Autodesk Fusion 360 part; units mm, degrees
(part 3 of 4)
  spline S1 degree 5 poles (46.7219, 69.0368) (46.744, 69.0368) (46.7882, 69.0364) (46.8546, 69.0344) (46.9431, 69.0291) (47.0539, 69.0189) (47.1646, 69.0061) (47.2752, 68.9921) (47.3856, 68.9776) (47.4957, 68.9631) (47.6056, 68.9482) (47.7152, 68.9327) (47.8246, 68.9161) (47.9339, 68.898) (48.043, 68.8784) (48.152, 68.8576) (48.2609, 68.8359) (48.3697, 68.8134) (48.4783, 68.7905) (48.5868, 68.7667) (48.6949, 68.742) (48.8027, 68.7157) (48.9099, 68.6877) (49.0166, 68.6578) (49.1229, 68.6261) (49.2287, 68.5929) (49.3342, 68.5585) (49.4395, 68.5233) (49.5445, 68.4876) (49.6493, 68.4511) (49.7537, 68.4138) (49.8576, 68.3753) (49.961, 68.3353) (50.0637, 68.2936) (50.1658, 68.2503) (50.2671, 68.2053) (50.3679, 68.159) (50.4681, 68.1114) (50.5678, 68.0629) (50.667, 68.0133) (50.7656, 67.9628) (50.8638, 67.9113) (50.9613, 67.8586) (51.0583, 67.8047) (51.1545, 67.7494) (51.2499, 67.6928) (51.3444, 67.6346) (51.438, 67.575) (51.5307, 67.5139) (51.6224, 67.4515) (51.7133, 67.3878) (51.8034, 67.3231) (51.8928, 67.2574) (51.9817, 67.1909) (52.07, 67.1238) (52.1579, 67.0561) (52.2454, 66.9877) (52.3323, 66.9187) (52.4188, 66.849) (52.5045, 66.7785) (52.5894, 66.707) (52.6733, 66.6343) (52.7562, 66.5605) (52.8379, 66.4854) (52.9186, 66.4092) (52.9985, 66.3321) (53.0777, 66.2544) (53.1565, 66.176) (53.2347, 66.0972) (53.3124, 66.0177) (53.3892, 65.9375) (53.4649, 65.8564) (53.5393, 65.7741) (53.6123, 65.6905) (53.684, 65.6058) (53.7546, 65.5202) (53.8243, 65.4337) (53.8933, 65.3467) (53.9617, 65.2592) (54.0293, 65.1712) (54.0961, 65.0826) (54.1618, 64.9932) (54.2262, 64.9028) (54.2891, 64.8115) (54.3506, 64.7192) (54.411, 64.626) (54.4703, 64.5322) (54.5289, 64.4379) (54.5866, 64.3432) (54.6436, 64.248) (54.6995, 64.1522) (54.7542, 64.0558) (54.8075, 63.9585) (54.8592, 63.8604) (54.9096, 63.7616) (54.9587, 63.6621) (55.0069, 63.5621) (55.0542, 63.4617) (55.1009, 63.3611) (55.1469, 63.2602) (55.192, 63.159) (55.236, 63.0573) (55.2787, 62.955) (55.3201, 62.8521) (55.3602, 62.7487) (55.399, 62.6447) (55.4367, 62.5404) (55.4734, 62.4357) (55.5094, 62.3308) (55.5446, 62.2257) (55.579, 62.1203) (55.6128, 62.0147) (55.6463, 61.9089) (55.6802, 61.8032) (55.7155, 61.698) (55.7535, 61.5938) (55.7954, 61.4912) (55.8424, 61.3909) (55.8953, 61.2935) (55.9545, 61.1995) (56.0198, 61.1093) (56.0911, 61.0234) (56.1677, 60.9421) (56.2492, 60.8658) (56.335, 60.7948) (56.4249, 60.7292) (56.5184, 60.6692) (56.6151, 60.6148) (56.7146, 60.5659) (56.8165, 60.522) (56.9203, 60.4826) (57.0255, 60.447) (57.1317, 60.4143) (57.2385, 60.3836) (57.3454, 60.3539) (57.4522, 60.3241) (57.5587, 60.2934) (57.6647, 60.261) (57.77, 60.2265) (57.8747, 60.1898) (57.9786, 60.151) (58.082, 60.1103) (58.1847, 60.0683) (58.2869, 60.025) (58.3886, 59.9809) (58.4898, 59.9358) (58.5907, 59.89) (58.6912, 59.8432) (58.7913, 59.7956) (58.8911, 59.7472) (58.9906, 59.6981) (59.0898, 59.6481) (59.1886, 59.5974) (59.2869, 59.5458) (59.3846, 59.4932) (59.4815, 59.4394) (59.5776, 59.384) (59.6727, 59.3271) (59.7668, 59.2686) (59.8601, 59.2086) (59.9527, 59.1475) (60.0447, 59.0854) (60.1363, 59.0227) (60.2275, 58.9593) (60.3182, 58.8952) (60.408, 58.8301) (60.4969, 58.7637) (60.5846, 58.6958) (60.671, 58.6263) (60.7563, 58.5554) (60.8407, 58.4833) (60.9244, 58.4104) (61.0078, 58.3369) (61.0907, 58.263) (61.1732, 58.1886) (61.2549, 58.1134) (61.3355, 58.0371) (61.4148, 57.9595) (61.4926, 57.8805) (61.5692, 57.8002) (61.6448, 57.7189) (61.7196, 57.6368) (61.7939, 57.5542) (61.868, 57.4714) (61.9414, 57.3881) (62.0141, 57.3042) (62.0857, 57.2193) (62.1557, 57.1334) (62.2242, 57.0461) (62.2911, 56.9576) (62.3567, 56.868) (62.4212, 56.7776) (62.485, 56.6867) (62.548, 56.5953) (62.6104, 56.5034) (62.6717, 56.411) (62.7319, 56.3178) (62.7906, 56.2237) (62.8478, 56.1287) (62.9035, 56.0327) (62.9579, 55.936) (63.0112, 55.8387) (63.0638, 55.741) (63.1157, 55.643) (63.1669, 55.5448) (63.2174, 55.4461) (63.2669, 55.347) (63.3153, 55.2472) (63.3623, 55.1468) (63.4079, 55.0456) (63.452, 54.9438) (63.4946, 54.8413) (63.5358, 54.7383) (63.5757, 54.6349) (63.6146, 54.5311) (63.6527, 54.427) (63.6901, 54.3227) (63.7269, 54.2181) (63.7631, 54.1132) (63.7982, 54.0079) (63.832, 53.9022) (63.8641, 53.796) (63.894, 53.6892) (63.9217, 53.5819) (63.9475, 53.474) (63.9717, 53.3657) (63.9947, 53.2571) (64.0171, 53.1484) (64.039, 53.0396) (64.0604, 52.9307) (64.0811, 52.8217) (64.1009, 52.7126) (64.1193, 52.6032) (64.1362, 52.4936) (64.1516, 52.3838) (64.1657, 52.2737) (64.1787, 52.1635) (64.1908, 52.0532) (64.2021, 51.9428) (64.2127, 51.8323) (64.2225, 51.7217) (64.2314, 51.611) (64.239, 51.5002) (64.2451, 51.3893) (64.2493, 51.2783) (64.2514, 51.1672) (64.2511, 51.0562) (64.2484, 50.9452) (64.2435, 50.8344) (64.2367, 50.7236) (64.2288, 50.6129) (64.2204, 50.5022) (64.2119, 50.3915) (64.2035, 50.2807) (64.195, 50.17) (64.1859, 50.0593) (64.1756, 49.9488) (64.1635, 49.8385) (64.1493, 49.7285) (64.1329, 49.6187) (64.1147, 49.5092) (64.0951, 49.3999) (64.0745, 49.2908) (64.0531, 49.1818) (64.0311, 49.073) (64.0084, 48.9644) (63.9846, 48.856) (63.9597, 48.748) (63.9332, 48.6402) (63.9052, 48.5328) (63.8756, 48.4259) (63.8445, 48.3194) (63.8118, 48.2135) (63.7778, 48.1079) (63.7427, 48.0028) (63.7065, 47.898) (63.6695, 47.7935) (63.6318, 47.6892) (63.5932, 47.5852) (63.5537, 47.4816) (63.513, 47.3784) (63.4708, 47.2758) (63.4271, 47.1739) (63.3816, 47.0727) (63.3346, 46.9722) (63.2863, 46.8723) (63.2368, 46.7729) (63.1866, 46.6739) (63.1356, 46.5753) (63.0839, 46.4771) (63.0314, 46.3793) (62.978, 46.2822) (62.9234, 46.1856) (62.8676, 46.0898) (62.8107, 45.9946) (62.7527, 45.9001) (62.6937, 45.8062) (62.6338, 45.7127) (62.573, 45.6198) (62.5112, 45.5276) (62.4483, 45.4361) (62.3842, 45.3456) (62.3186, 45.2561) (62.2515, 45.1677) (62.1831, 45.0803) (62.1136, 44.9938) (62.0431, 44.908) (61.9718, 44.8228) (61.8997, 44.7383) (61.8267, 44.6547) (61.7525, 44.572) (61.6771, 44.4907) (61.6004, 44.4105) (61.5227, 44.3311) (61.445, 44.2518) (61.3683, 44.1715) (61.2938, 44.0892) (61.2229, 44.0038) (61.1565, 43.9146) (61.0957, 43.8215) (61.0409, 43.7246) (60.9925, 43.6242) (60.9507, 43.521) (60.9156, 43.4154) (60.8872, 43.3079) (60.8653, 43.1989) (60.8499, 43.0889) (60.8409, 42.9781) (60.8381, 42.8669) (60.8415, 42.7557) (60.851, 42.6449) (60.8662, 42.5348) (60.8867, 42.4256) (60.9115, 42.3173) (60.9392, 42.2098) (60.968, 42.1026) (60.9964, 41.9954) (61.023, 41.8879) (61.047, 41.7797) (61.0685, 41.671) (61.0879, 41.5617) (61.106, 41.452) (61.1236, 41.3423) (61.141, 41.2325) (61.1582, 41.1228) (61.1746, 41.013) (61.1896, 40.9031) (61.2024, 40.793) (61.2128, 40.6826) (61.2208, 40.5719) (61.2269, 40.461) (61.2316, 40.3499) (61.2355, 40.2389) (61.239, 40.1278) (61.2421, 40.0168) (61.2445, 39.9058) (61.246, 39.7949) (61.2462, 39.6839) (61.2449, 39.573) (61.2421, 39.462) (61.2379, 39.351) (61.2325, 39.2401) (61.226, 39.1292) (61.2187, 39.0184) (61.2105, 38.9078) (61.2013, 38.7971) (61.1911, 38.6866) (61.1797, 38.5762) (61.1669, 38.466) (61.1527, 38.3559) (61.1368, 38.246) (61.1194, 38.1363) (61.1004, 38.0269) (61.0798, 37.9179) (61.0578, 37.8092) (61.0344, 37.7008) (61.0096, 37.5927) (60.9836, 37.4848) (60.9564, 37.3773) (60.928, 37.27) (60.8983, 37.1631) (60.8673, 37.0566) (60.8349, 36.9505) (60.8013, 36.8449) (60.7664, 36.7397) (60.7305, 36.6348) (60.6937, 36.5302) (60.6561, 36.4258) (60.6176, 36.3218) (60.5782, 36.2181) (60.5377, 36.1148) (60.4958, 36.0121) (60.4524, 35.9101) (60.4074, 35.8088) (60.361, 35.7081) (60.3132, 35.6081) (60.2643, 35.5086) (60.2146, 35.4095) (60.1642, 35.3108) (60.113, 35.2125) (60.061, 35.1145) (60.0081, 35.0171) (59.954, 34.9203) (59.8987, 34.8242) (59.842, 34.7288) (59.784, 34.6342) (59.7248, 34.5403) (59.6643, 34.4473) (59.6026, 34.355) (59.5397, 34.2635) (59.4757, 34.1728) (59.4105, 34.083) (59.3442, 33.994) (59.2768, 33.9058) (59.2083, 33.8185) (59.1388, 33.732) (59.0682, 33.6463) (58.9966, 33.5614) (58.9242, 33.4773) (58.8509, 33.394) (58.7768, 33.3113) (58.7018, 33.2294) (58.6261, 33.1482) (58.5496, 33.0677) (58.4723, 32.988) (58.3941, 32.9092) (58.315, 32.8314) (58.2349, 32.7545) (58.1538, 32.6787) (58.0717, 32.6039) (57.9887, 32.5302) (57.9048, 32.4575) (57.82, 32.3858) (57.7344, 32.3151) (57.6479, 32.2455) (57.5605, 32.177) (57.4723, 32.1096) (57.3832, 32.0435) (57.2934, 31.9785) (57.2027, 31.9146) (57.1115, 31.8514) (57.0198, 31.7889) (56.9277, 31.727) (56.8352, 31.6656) (56.7422, 31.605) (56.6487, 31.5453) (56.5544, 31.4868) (56.4594, 31.4297) (56.3634, 31.3742) (56.2666, 31.3202) (56.1691, 31.2675) (56.071, 31.2158) (55.9724, 31.165) (55.8735, 31.1149) (55.7742, 31.0657) (55.6743, 31.0176) (55.5738, 30.9708) (55.4727, 30.9256) (55.3707, 30.8821) (55.268, 30.8403) (55.1647, 30.7999) (55.0609, 30.7608) (54.9568, 30.7227) (54.8524, 30.6853) (54.7478, 30.6484) (54.643, 30.612) (54.5382, 30.576) (54.4331, 30.5405) (54.3277, 30.5058) (54.2221, 30.472) (54.116, 30.4396) (54.0094, 30.4089) (53.9022, 30.3803) (53.7945, 30.3537) (53.6863, 30.3292) (53.5777, 30.3064) (53.4688, 30.2852) (53.3596, 30.2651) (53.2504, 30.2459) (53.141, 30.2274) (53.0315, 30.2097) (52.9218, 30.1927) (52.812, 30.1767) (52.702, 30.1617) (52.5918, 30.1482) (52.4813, 30.1362) (52.3708, 30.1261) (52.2601, 30.1179) (52.1493, 30.1117) (52.0384, 30.1071) (51.9274, 30.1038) (51.8164, 30.1015) (51.7053, 30.0998) (51.5943, 30.0988) (51.4832, 30.0986) (51.3721, 30.0996) (51.2612, 30.102) (51.1503, 30.1063) (51.0396, 30.1124) (50.9289, 30.1203) (50.8183, 30.1293) (50.7077, 30.1392) (50.5971, 30.1495) (50.4865, 30.1602) (50.3761, 30.1715) (50.2658, 30.1842) (50.1558, 30.1989) (50.0462, 30.2162) (49.9371, 30.2363) (49.8284, 30.2591) (49.7203, 30.2841) (49.6126, 30.3107) (49.5052, 30.3382) (49.3979, 30.3658) (49.2906, 30.393) (49.183, 30.4195) (49.075, 30.4448) (48.9663, 30.4684) (48.8569, 30.4893) (48.7469, 30.5065) (48.6363, 30.5186) (48.5256, 30.5242) (48.4148, 30.5224) (48.3045, 30.5124) (48.195, 30.4943) (48.0865, 30.4685) (47.9797, 30.4359) (47.8747, 30.3971) (47.7721, 30.353) (47.6723, 30.3037) (47.5755, 30.2494) (47.482, 30.1902) (47.3918, 30.1263) (47.3048, 30.058) (47.2205, 29.986) (47.1382, 29.9113) (47.0572, 29.835) (46.9768, 29.758) (46.8963, 29.6812) (46.8152, 29.6052) (46.7333, 29.5304) (46.6504, 29.4567) (46.5663, 29.3844) (46.4812, 29.3132) (46.3951, 29.2433) (46.308, 29.1744) (46.2201, 29.1066) (46.1313, 29.0398) (46.0419, 28.974) (45.9517, 28.9092) (45.8608, 28.8456) (45.7691, 28.7831) (45.6767, 28.7218) (45.5834, 28.6618) (45.4894, 28.6029) (45.3947, 28.5451) (45.2994, 28.4883) (45.2035, 28.4325) (45.107, 28.3777) (45.01, 28.3239) (44.9123, 28.2714) (44.814, 28.2203) (44.7151, 28.1705) (44.6154, 28.1221) (44.5152, 28.0749) (44.4145, 28.0287) (44.3134, 27.9832) (44.212, 27.9383) (44.1103, 27.8939) (44.0084, 27.8502) (43.906, 27.8074) (43.8032, 27.766) (43.6997, 27.7262) (43.5956, 27.6882) (43.4909, 27.6518) (43.3856, 27.6169) (43.28, 27.5832) (43.174, 27.5504) (43.0678, 27.5185) (42.9613, 27.4875) (42.8545, 27.4576) (42.7474, 27.429) (42.6398, 27.402) (42.5318, 27.3767) (42.4234, 27.3531) (42.3146, 27.3311) (42.2056, 27.3106) (42.0963, 27.2912) (41.9869, 27.2727) (41.8775, 27.255) (41.7679, 27.2376) (41.6583, 27.2207) (41.5486, 27.2041) (41.4387, 27.1881) (41.3286, 27.173) (41.2184, 27.1594) (41.1081, 27.1478) (40.9975, 27.1384) (40.8868, 27.1314) (40.7759, 27.1266) (40.6649, 27.1235) (40.5538, 27.1216) (40.4427, 27.1205) (40.3316, 27.1199) (40.2205, 27.12) (40.1095, 27.1209) (39.9986, 27.1232) (39.8877, 27.1272) (39.7769, 27.1331) (39.6662, 27.1408) (39.5556, 27.15) (39.4451, 27.1603) (39.3346, 27.1714) (39.2242, 27.1832) (39.1139, 27.1956) (39.0036, 27.2088) (38.8936, 27.2231) (38.7837, 27.2389) (38.6741, 27.2563) (38.5647, 27.2754) (38.4557, 27.2963) (38.347, 27.3188) (38.2386, 27.3427) (38.1306, 27.3679) (38.0228, 27.394) (37.9152, 27.4209) (37.8078, 27.4484) (37.7004, 27.4764) (37.5932, 27.505) (37.4863, 27.5344) (37.3796, 27.565) (37.2735, 27.5972) (37.168, 27.6313) (37.0632, 27.6673) (36.959, 27.7053) (36.8555, 27.745) (36.7524, 27.7861) (36.6498, 27.8282) (36.5475, 27.8712) (36.4455, 27.915) (36.344, 27.9596) (36.2429, 28.0052) (36.1423, 28.0518) (36.0423, 28.0997) (35.9429, 28.1489) (35.8441, 28.1993) (35.7459, 28.2509) (35.6483, 28.3035) (35.5512, 28.3571) (35.4546, 28.4116) (35.3585, 28.4669) (35.2627, 28.523) (35.1674, 28.5799) (35.0726, 28.6376) (34.9785, 28.6964) (34.8851, 28.7564) (34.7927, 28.8178) (34.7013, 28.8807) (34.611, 28.9451) (34.5217, 29.0109) (34.4332, 29.078) (34.3456, 29.1461) (34.2585, 29.215) (34.172, 29.2846) (34.086, 29.3549) (34.0008, 29.4261) (33.9165, 29.4983) (33.8332, 29.5716) (33.7509, 29.6461) (33.6697, 29.7218) (33.5895, 29.7986) (33.5103, 29.8764) (33.4318, 29.955) (33.3541, 30.0343) (33.2772, 30.1144) (33.201, 30.1951) (33.1257, 30.2767) (33.0514, 30.3591) (32.9781, 30.4425) (32.9059, 30.5268) (32.8348, 30.6121) (32.7648, 30.6983) (32.696, 30.7855) (32.6283, 30.8735) (32.5617, 30.9622) (32.4961, 31.0518) (32.4315, 31.142) (32.3679, 31.233) (32.3053, 31.3246) (32.2437, 31.4168) (32.1831, 31.5098) (32.1237, 31.6035) (32.0655, 31.698) (32.0086, 31.7933) (31.9529, 31.8893) (31.8987, 31.9861) (31.8457, 32.0836) (31.794, 32.1818) (31.7435, 32.2806) (31.6941, 32.3799) (31.6455, 32.4796) (31.5977, 32.5796) (31.5505, 32.68) (31.5038, 32.7805) (31.4578, 32.8814) (31.4125, 32.9826) (31.3681, 33.0843) (31.3249, 33.1866) (31.2832, 33.2895) (31.2432, 33.3931) (31.2053, 33.4974) (31.1696, 33.6025) (31.1361, 33.7081) (31.1044, 33.8143) (31.0739, 33.9209) (31.0439, 34.0277) (31.0133, 34.1343) (30.9811, 34.2406) (30.9464, 34.3461) (30.9083, 34.4505) (30.866, 34.5533) (30.8192, 34.6539) (30.7675, 34.752) (30.7105, 34.8472) (30.6482, 34.939) (30.5807, 35.0273) (30.5081, 35.1116) (30.4306, 35.1918) (30.3484, 35.2673) (30.2618, 35.3377) (30.1712, 35.4024) (30.0768, 35.461) (29.979, 35.5134) (29.8783, 35.5598) (29.7752, 35.6007) (29.6703, 35.6372) (29.5642, 35.6702) (29.4573, 35.7012) (29.3503, 35.7312) (29.2435, 35.7612) (29.137, 35.7921) (29.0311, 35.8245) (28.9258, 35.8588) (28.8212, 35.8952) (28.7172, 35.9336) (28.6138, 35.9738) (28.511, 36.0156) (28.4087, 36.0586) (28.3068, 36.1025) (28.2053, 36.1473) (28.1042, 36.1928) (28.0035, 36.2392) (27.9033, 36.2865) (27.8036, 36.3348) (27.7044, 36.3842) (27.6058, 36.4349) (27.5078, 36.4868) (27.4106, 36.5399) (27.3139, 36.5943) (27.2179, 36.6499) (27.1225, 36.7064) (27.0275, 36.7638) (26.933, 36.822) (26.8389, 36.8809) (26.7453, 36.9406) (26.6524, 37.0012) (26.5602, 37.063) (26.4688, 37.126) (26.3784, 37.1904) (26.289, 37.256) (26.2003, 37.3228) (26.1125, 37.3907) (26.0254, 37.4595) (25.9389, 37.5292) (25.8532, 37.5997) (25.7682, 37.6711) (25.6839, 37.7434) (25.6006, 37.8168) (25.5182, 37.8912) (25.4368, 37.9666) (25.3563, 38.0431) (25.2767, 38.1205) (25.1981, 38.1989) (25.1202, 38.2781) (25.0433, 38.3581) (24.9672, 38.4389) (24.8919, 38.5205) (24.8174, 38.6028) (24.7437, 38.6858) (24.6709, 38.7696) (24.5988, 38.854) (24.5276, 38.9392) (24.4572, 39.0251) (24.3877, 39.1117) (24.3193, 39.1992) (24.252, 39.2875) (24.1859, 39.3766) (24.1211, 39.4667) (24.0577, 39.5577) (23.9954, 39.6496) (23.9343, 39.7421) (23.8741, 39.8353) (23.8148, 39.9291) (23.7563, 40.0234) (23.6988, 40.1182) (23.6425, 40.2137) (23.5874, 40.31) (23.5337, 40.407) (23.4816, 40.505) (23.4309, 40.6037) (23.3815, 40.7031) (23.3332, 40.803) (23.2857, 40.9033) (23.2391, 41.004) (23.1933, 41.105) (23.1486, 41.2064) (23.105, 41.3083) (23.0626, 41.4107) (23.0216, 41.5136) (22.9817, 41.6171) (22.9427, 41.7209) (22.9045, 41.8251) (22.8669, 41.9295) (22.8299, 42.0342) (22.7938, 42.1391) (22.7591, 42.2444) (22.726, 42.3502) (22.6951, 42.4566) (22.6663, 42.5637) (22.6396, 42.6713) (22.6146, 42.7794) (22.5909, 42.8879) (22.568, 42.9966) (22.5459, 43.1053) (22.5245, 43.2142) (22.5039, 43.3232) (22.4846, 43.4324) (22.4667, 43.5418) (22.4504, 43.6515) (22.4359, 43.7615) (22.4229, 43.8717) (22.4113, 43.9821) (22.4009, 44.0926) (22.3914, 44.2032) (22.3826, 44.3138) (22.3747, 44.4246) (22.3674, 44.5353) (22.361, 44.6462) (22.3557, 44.7572) (22.3519, 44.8682) (22.3499, 44.9792) (22.3499, 45.0903) (22.3523, 45.2012) (22.3569, 45.3121) (22.3632, 45.4229) (22.3708, 45.5337) (22.3789, 45.6444) (22.3871, 45.7551) (22.3951, 45.8659) (22.4031, 45.9766) (22.4116, 46.0873) (22.4211, 46.1979) (22.4323, 46.3083) (22.4457, 46.4185) (22.4613, 46.5285) (22.4791, 46.6381) (22.499, 46.7473) (22.5206, 46.8562) (22.5436, 46.9648) (22.5677, 47.0731) (22.5928, 47.1812) (22.6186, 47.289) (22.6451, 47.3967) (22.6723, 47.5043) (22.7004, 47.6116) (22.7294, 47.7187) (22.7597, 47.8254) (22.7914, 47.9318) (22.8246, 48.0376) (22.8594, 48.1429) (22.8956, 48.2478) (22.9333, 48.3521) (22.9722, 48.4559) (23.0123, 48.5593) (23.0535, 48.6623) (23.0957, 48.7648) (23.139, 48.8669) (23.1834, 48.9686) (23.2289, 49.0698) (23.2756, 49.1704) (23.3236, 49.2705) (23.3729, 49.3699) (23.4236, 49.4685) (23.4757, 49.5665) (23.5289, 49.6638) (23.5833, 49.7604) (23.6386, 49.8565) (23.6947, 49.9522) (23.7516, 50.0474) (23.8092, 50.1422) (23.8677, 50.2364) (23.9272, 50.3301) (23.9877, 50.4231) (24.0495, 50.5152) (24.1126, 50.6065) (24.1771, 50.6969) (24.2429, 50.7863) (24.3099, 50.8747) (24.3781, 50.9623) (24.4471, 51.0492) (24.5168, 51.1355) (24.587, 51.2215) (24.6576, 51.3072) (24.7287, 51.3924) (24.8006, 51.4769) (24.8738, 51.5603) (24.9487, 51.6423) (25.0254, 51.7227) (25.1034, 51.802) (25.1817, 51.881) (25.2591, 51.9608) (25.3339, 52.0428) (25.4046, 52.128) (25.4701, 52.2173) (25.5299, 52.3108) (25.5835, 52.4083) (25.6312, 52.5092) (25.6729, 52.6128) (25.7087, 52.7186) (25.7384, 52.8259) (25.7617, 52.9345) (25.7784, 53.0441) (25.788, 53.1545) (25.7907, 53.2654) (25.7868, 53.3765) (25.7767, 53.4874) (25.7614, 53.5977) (25.7416, 53.7074) (25.7185, 53.8161) (25.693, 53.9242) (25.6661, 54.0317) (25.6387, 54.139) (25.6117, 54.2465) (25.5859, 54.3543) (25.5618, 54.4626) (25.5399, 54.5714) (25.5201, 54.6807) (25.5027, 54.7904) (25.4873, 54.9003) (25.4735, 55.0104) (25.4607, 55.1207) (25.4484, 55.231) (25.4361, 55.3413) (25.4238, 55.4516) (25.4118, 55.562) (25.4007, 55.6725) (25.3913, 55.783) (25.384, 55.8937) (25.3792, 56.0045) (25.3766, 56.1155) (25.3758, 56.2265) (25.3762, 56.3376) (25.3772, 56.4487) (25.3786, 56.5599) (25.3805, 56.6709) (25.3834, 56.7819) (25.3877, 56.8928) (25.3941, 57.0035) (25.4027, 57.1141) (25.4136, 57.2246) (25.4264, 57.3349) (25.4407, 57.4451) (25.456, 57.5551) (25.4719, 57.6649) (25.4881, 57.7747) (25.5045, 57.8843) (25.5213, 57.994) (25.5387, 58.1035) (25.5568, 58.213) (25.5763, 58.3223) (25.5973, 58.4313) (25.6204, 58.5398) (25.6456, 58.6478) (25.6731, 58.7552) (25.7025, 58.8621) (25.7334, 58.9686) (25.7655, 59.0748) (25.7982, 59.1808) (25.8314, 59.2867) (25.8652, 59.3923) (25.8998, 59.4977) (25.9357, 59.6025) (25.9732, 59.7068) (26.0123, 59.8105) (26.0531, 59.9136) (26.0951, 60.0162) (26.1381, 60.1185) (26.1816, 60.2205) (26.2257, 60.3224) (26.2703, 60.424) (26.3157, 60.5252) (26.3624, 60.6258) (26.4105, 60.7257) (26.4603, 60.8247) (26.5118, 60.9229) (26.5648, 61.0204) (26.6191, 61.1172) (26.6744, 61.2135) (26.7305, 61.3092) (26.7875, 61.4045) (26.8454, 61.4991) (26.9043, 61.5931) (26.9645, 61.6863) (27.0259, 61.7787) (27.0886, 61.8702) (27.1525, 61.9609) (27.2176, 62.0508) (27.2838, 62.1399) (27.351, 62.2283) (27.4192, 62.3159) (27.4886, 62.4026) (27.559, 62.4884) (27.6306, 62.5732) (27.7034, 62.657) (27.7772, 62.7399) (27.852, 62.8219) (27.9277, 62.9032) (28.0041, 62.9838) (28.0811, 63.0637) (28.1588, 63.1431) (28.237, 63.2218) (28.316, 63.2999) (28.3957, 63.3771) (28.4762, 63.4536) (28.5576, 63.529) (28.64, 63.6035) (28.7234, 63.6768) (28.8079, 63.7489) (28.8933, 63.8198) (28.9798, 63.8893) (29.0673, 63.9577) (29.1557, 64.0248) (29.245, 64.0907) (29.3351, 64.1555) (29.4258, 64.2194) (29.5171, 64.2824) (29.6089, 64.3447) (29.7011, 64.4063) (29.7938, 64.4674) (29.8869, 64.5277) (29.9804, 64.5873) (30.0746, 64.646) (30.1694, 64.7036) (30.2649, 64.7601) (30.3611, 64.8152) (30.4582, 64.8688) (30.5561, 64.9208) (30.6549, 64.9713) (30.7543, 65.0202) (30.8545, 65.0677) (30.9552, 65.114) (31.0564, 65.1592) (31.158, 65.2037) (31.2599, 65.2473) (31.3622, 65.2902) (31.4649, 65.3321) (31.568, 65.3728) (31.6716, 65.4124) (31.7757, 65.4507) (31.8802, 65.4877) (31.9851, 65.5236) (32.0903, 65.5585) (32.1958, 65.5926) (32.3015, 65.6259) (32.4075, 65.6583) (32.5139, 65.6897) (32.6206, 65.7198) (32.7277, 65.7485) (32.8353, 65.7757) (32.9433, 65.8011) (33.0517, 65.8248) (33.1605, 65.8467) (33.2696, 65.8671) (33.3788, 65.8861) (33.4883, 65.904) (33.5979, 65.9209) (33.7076, 65.9372) (33.8175, 65.9529) (33.9274, 65.968) (34.0376, 65.9821) (34.1478, 65.9948) (34.2583, 66.0057) (34.3689, 66.0144) (34.4797, 66.0206) (34.5907, 66.0247) (34.7017, 66.0268) (34.8128, 66.0276) (34.9238, 66.0275) (35.0349, 66.0269) (35.1459, 66.026) (35.2568, 66.025) (35.3678, 66.0237) (35.4789, 66.0219) (35.5899, 66.0193) (35.7009, 66.0155) (35.8118, 66.0102) (35.9226, 66.0029) (36.0331, 65.9934) (36.1434, 65.9817) (36.2536, 65.9679) (36.3635, 65.9525) (36.4733, 65.9357) (36.583, 65.9178) (36.6925, 65.8988) (36.8016, 65.8783) (36.9103, 65.8557) (37.0183, 65.8306) (37.1257, 65.8028) (37.2324, 65.7727) (37.3389, 65.7414) (37.4454, 65.7104) (37.5526, 65.6817) (37.6607, 65.6569) (37.7699, 65.6374) (37.8802, 65.6239) (37.9913, 65.6168) (38.1028, 65.6159) (38.2143, 65.6211) (38.3253, 65.6322) (38.4353, 65.6492) (38.5439, 65.6724) (38.6508, 65.7019) (38.7557, 65.738) (38.8582, 65.7806) (38.9579, 65.8295) (39.0546, 65.8844) (39.1481, 65.9446) (39.2383, 66.0096) (39.3255, 66.0785) (39.4099, 66.1506) (39.4923, 66.2249) (39.5732, 66.3008) (39.6534, 66.3774) (39.7336, 66.4541) (39.8142, 66.5305) (39.8954, 66.6062) (39.9776, 66.6808) (40.0609, 66.7543) (40.1453, 66.8265) (40.2307, 66.8975) (40.3171, 66.9672) (40.4043, 67.0359) (40.4923, 67.1035) (40.5811, 67.1701) (40.6704, 67.2359) (40.7603, 67.3008) (40.8509, 67.365) (40.9421, 67.4283) (41.034, 67.4906) (41.1266, 67.5518) (41.22, 67.6117) (41.3144, 67.6701) (41.4096, 67.727) (41.5056, 67.7824) (41.6024, 67.8364) (41.6997, 67.8894) (41.7975, 67.9416) (41.8956, 67.9932) (41.9941, 68.0443) (42.0929, 68.0946) (42.1923, 68.1438) (42.2924, 68.1915) (42.3933, 68.2373) (42.4951, 68.281) (42.5978, 68.3228) (42.7011, 68.363) (42.805, 68.4019) (42.9092, 68.44) (43.0137, 68.4773) (43.1184, 68.5139) (43.2234, 68.5497) (43.3287, 68.5843) (43.4344, 68.6175) (43.5407, 68.6492) (43.6474, 68.6793) (43.7546, 68.708) (43.8621, 68.7355) (43.9699, 68.7619) (44.078, 68.7874) (44.1863, 68.8118) (44.2948, 68.835) (44.4035, 68.8568) (44.5126, 68.8771) (44.6219, 68.8958) (44.7315, 68.9131) (44.8414, 68.929) (44.9515, 68.9438) (45.0617, 68.9575) (45.1721, 68.9699) (45.2826, 68.9807) (45.3933, 68.9894) (45.5042, 68.9957) (45.6151, 68.9995) (45.7262, 69.0011) (45.8374, 69.0015) (45.9485, 69.002) (46.0594, 69.0038) (46.1701, 69.0079) (46.2806, 69.0143) (46.391, 69.0221) (46.5012, 69.0298) (46.5894, 69.0345) (46.6556, 69.0364) (46.6998, 69.0368) (46.7219, 69.0368) knots 0 0 0 0 0 0 0.00082645 0.00165289 0.00247934 0.00330579 0.00413223 0.00495868 0.00578512 0.00661157 0.00743802 0.00826446 0.00909091 0.00991736 0.0107438 0.01157025 0.01239669 0.01322314 0.01404959 0.01487603 0.01570248 0.01652893 0.01735537 0.01818182 0.01900826 0.01983471 0.02066116 0.0214876 0.02231405 0.0231405 0.02396694 0.02479339 0.02561983 0.02644628 0.02727273 0.02809917 0.02892562 0.02975207 0.03057851 0.03140496 0.0322314 0.03305785 0.0338843 0.03471074 0.03553719 0.03636364 0.03719008 0.03801653 0.03884298 0.03966942 0.04049587 0.04132231 0.04214876 0.04297521 0.04380165 0.0446281 0.04545455 0.04628099 0.04710744 0.04793388 0.04876033 0.04958678 0.05041322 0.05123967 0.05206612 0.05289256 0.05371901 0.05454545 0.0553719 0.05619835 0.05702479 0.05785124 0.05867769 0.05950413 0.06033058 0.06115702 0.06198347 0.06280992 0.06363636 0.06446281 0.06528926 0.0661157 0.06694215 0.0677686 0.06859504 0.06942149 0.07024793 0.07107438 0.07190083 0.07272727 0.07355372 0.07438017 0.07520661 0.07603306 0.0768595 0.07768595 0.0785124 0.07933884 0.08016529 0.08099174 0.08181818 0.08264463 0.08347107 0.08429752 0.08512397 0.08595041 0.08677686 0.08760331 0.08842975 0.0892562 0.09008264 0.09090909 0.09173554 0.09256198 0.09338843 0.09421488 0.09504132 0.09586777 0.09669421 0.09752066 0.09834711 0.09917355 0.1 0.10082645 0.10165289 0.10247934 0.10330579 0.10413223 0.10495868 0.10578512 0.10661157 0.10743802 0.10826446 0.10909091 0.10991736 0.1107438 0.11157025 0.11239669 0.11322314 0.11404959 0.11487603 0.11570248 0.11652893 0.11735537 0.11818182 0.11900826 0.11983471 0.12066116 0.1214876 0.12231405 0.1231405 0.12396694 0.12479339 0.12561983 0.12644628 0.12727273 0.12809917 0.12892562 0.12975207 0.13057851 0.13140496 0.1322314 0.13305785 0.1338843 0.13471074 0.13553719 0.13636364 0.13719008 0.13801653 0.13884298 0.13966942 0.14049587 0.14132231 0.14214876 0.14297521 0.14380165 0.1446281 0.14545455 0.14628099 0.14710744 0.14793388 0.14876033 0.14958678 0.15041322 0.15123967 0.15206612 0.15289256 0.15371901 0.15454545 0.1553719 0.15619835 0.15702479 0.15785124 0.15867769 0.15950413 0.16033058 0.16115702 0.16198347 0.16280992 0.16363636 0.16446281 0.16528926 0.1661157 0.16694215 0.1677686 0.16859504 0.16942149 0.17024793 0.17107438 0.17190083 0.17272727 0.17355372 0.17438017 0.17520661 0.17603306 0.1768595 0.17768595 0.1785124 0.17933884 0.18016529 0.18099174 0.18181818 0.18264463 0.18347107 0.18429752 0.18512397 0.18595041 0.18677686 0.18760331 0.18842975 0.1892562 0.19008264 0.19090909 0.19173554 0.19256198 0.19338843 0.19421488 0.19504132 0.19586777 0.19669421 0.19752066 0.19834711 0.19917355 0.2 0.20082645 0.20165289 0.20247934 0.20330579 0.20413223 0.20495868 0.20578512 0.20661157 0.20743802 0.20826446 0.20909091 0.20991736 0.2107438 0.21157025 0.21239669 0.21322314 0.21404959 0.21487603 0.21570248 0.21652893 0.21735537 0.21818182 0.21900826 0.21983471 0.22066116 0.2214876 0.22231405 0.2231405 0.22396694 0.22479339 0.22561983 0.22644628 0.22727273 0.22809917 0.22892562 0.22975207 0.23057851 0.23140496 0.2322314 0.23305785 0.2338843 0.23471074 0.23553719 0.23636364 0.23719008 0.23801653 0.23884298 0.23966942 0.24049587 0.24132231 0.24214876 0.24297521 0.24380165 0.2446281 0.24545455 0.24628099 0.24710744 0.24793388 0.24876033 0.24958678 0.25041322 0.25123967 0.25206612 0.25289256 0.25371901 0.25454545 0.2553719 0.25619835 0.25702479 0.25785124 0.25867769 0.25950413 0.26033058 0.26115702 0.26198347 0.26280992 0.26363636 0.26446281 0.26528926 0.2661157 0.26694215 0.2677686 0.26859504 0.26942149 0.27024793 0.27107438 0.27190083 0.27272727 0.27355372 0.27438017 0.27520661 0.27603306 0.2768595 0.27768595 0.2785124 0.27933884 0.28016529 0.28099174 0.28181818 0.28264463 0.28347107 0.28429752 0.28512397 0.28595041 0.28677686 0.28760331 0.28842975 0.2892562 0.29008264 0.29090909 0.29173554 0.29256198 0.29338843 0.29421488 0.29504132 0.29586777 0.29669421 0.29752066 0.29834711 0.29917355 0.3 0.30082645 0.30165289 0.30247934 0.30330579 0.30413223 0.30495868 0.30578512 0.30661157 0.30743802 0.30826446 0.30909091 0.30991736 0.3107438 0.31157025 0.31239669 0.31322314 0.31404959 0.31487603 0.31570248 0.31652893 0.31735537 0.31818182 0.31900826 0.31983471 0.32066116 0.3214876 0.32231405 0.3231405 0.32396694 0.32479339 0.32561983 0.32644628 0.32727273 0.32809917 0.32892562 0.32975207 0.33057851 0.33140496 0.3322314 0.33305785 0.3338843 0.33471074 0.33553719 0.33636364 0.33719008 0.33801653 0.33884298 0.33966942 0.34049587 0.34132231 0.34214876 0.34297521 0.34380165 0.3446281 0.34545455 0.34628099 0.34710744 0.34793388 0.34876033 0.34958678 0.35041322 0.35123967 0.35206612 0.35289256 0.35371901 0.35454545 0.3553719 0.35619835 0.35702479 0.35785124 0.35867769 0.35950413 0.36033058 0.36115702 0.36198347 0.36280992 0.36363636 0.36446281 0.36528926 0.3661157 0.36694215 0.3677686 0.36859504 0.36942149 0.37024793 0.37107438 0.37190083 0.37272727 0.37355372 0.37438017 0.37520661 0.37603306 0.3768595 0.37768595 0.3785124 0.37933884 0.38016529 0.38099174 0.38181818 0.38264463 0.38347107 0.38429752 0.38512397 0.38595041 0.38677686 0.38760331 0.38842975 0.3892562 0.39008264 0.39090909 0.39173554 0.39256198 0.39338843 0.39421488 0.39504132 0.39586777 0.39669421 0.39752066 0.39834711 0.39917355 0.4 0.40082645 0.40165289 0.40247934 0.40330579 0.40413223 0.40495868 0.40578512 0.40661157 0.40743802 0.40826446 0.40909091 0.40991736 0.4107438 0.41157025 0.41239669 0.41322314 0.41404959 0.41487603 0.41570248 0.41652893 0.41735537 0.41818182 0.41900826 0.41983471 0.42066116 0.4214876 0.42231405 0.4231405 0.42396694 0.42479339 0.42561983 0.42644628 0.42727273 0.42809917 0.42892562 0.42975207 0.43057851 0.43140496 0.4322314 0.43305785 0.4338843 0.43471074 0.43553719 0.43636364 0.43719008 0.43801653 0.43884298 0.43966942 0.44049587 0.44132231 0.44214876 0.44297521 0.44380165 0.4446281 0.44545455 0.44628099 0.44710744 0.44793388 0.44876033 0.44958678 0.45041322 0.45123967 0.45206612 0.45289256 0.45371901 0.45454545 0.4553719 0.45619835 0.45702479 0.45785124 0.45867769 0.45950413 0.46033058 0.46115702 0.46198347 0.46280992 0.46363636 0.46446281 0.46528926 0.4661157 0.46694215 0.4677686 0.46859504 0.46942149 0.47024793 0.47107438 0.47190083 0.47272727 0.47355372 0.47438017 0.47520661 0.47603306 0.4768595 0.47768595 0.4785124 0.47933884 0.48016529 0.48099174 0.48181818 0.48264463 0.48347107 0.48429752 0.48512397 0.48595041 0.48677686 0.48760331 0.48842975 0.4892562 0.49008264 0.49090909 0.49173554 0.49256198 0.49338843 0.49421488 0.49504132 0.49586777 0.49669421 0.49752066 0.49834711 0.49917355 0.5 0.50082645 0.50165289 0.50247934 0.50330579 0.50413223 0.50495868 0.50578512 0.50661157 0.50743802 0.50826446 0.50909091 0.50991736 0.5107438 0.51157025 0.51239669 0.51322314 0.51404959 0.51487603 0.51570248 0.51652893 0.51735537 0.51818182 0.51900826 0.51983471 0.52066116 0.5214876 0.52231405 0.5231405 0.52396694 0.52479339 0.52561983 0.52644628 0.52727273 0.52809917 0.52892562 0.52975207 0.53057851 0.53140496 0.5322314 0.53305785 0.5338843 0.53471074 0.53553719 0.53636364 0.53719008 0.53801653 0.53884298 0.53966942 0.54049587 0.54132231 0.54214876 0.54297521 0.54380165 0.5446281 0.54545455 0.54628099 0.54710744 0.54793388 0.54876033 0.54958678 0.55041322 0.55123967 0.55206612 0.55289256 0.55371901 0.55454545 0.5553719 0.55619835 0.55702479 0.55785124 0.55867769 0.55950413 0.56033058 0.56115702 0.56198347 0.56280992 0.56363636 0.56446281 0.56528926 0.5661157 0.56694215 0.5677686 0.56859504 0.56942149 0.57024793 0.57107438 0.57190083 0.57272727 0.57355372 0.57438017 0.57520661 0.57603306 0.5768595 0.57768595 0.5785124 0.57933884 0.58016529 0.58099174 0.58181818 0.58264463 0.58347107 0.58429752 0.58512397 0.58595041 0.58677686 0.58760331 0.58842975 0.5892562 0.59008264 0.59090909 0.59173554 0.59256198 0.59338843 0.59421488 0.59504132 0.59586777 0.59669421 0.59752066 0.59834711 0.59917355 0.6 0.60082645 0.60165289 0.60247934 0.60330579 0.60413223 0.60495868 0.60578512 0.60661157 0.60743802 0.60826446 0.60909091 0.60991736 0.6107438 0.61157025 0.61239669 0.61322314 0.61404959 0.61487603 0.61570248 0.61652893 0.61735537 0.61818182 0.61900826 0.61983471 0.62066116 0.6214876 0.62231405 0.6231405 0.62396694 0.62479339 0.62561983 0.62644628 0.62727273 0.62809917 0.62892562 0.62975207 0.63057851 0.63140496 0.6322314 0.63305785 0.6338843 0.63471074 0.63553719 0.63636364 0.63719008 0.63801653 0.63884298 0.63966942 0.64049587 0.64132231 0.64214876 0.64297521 0.64380165 0.6446281 0.64545455 0.64628099 0.64710744 0.64793388 0.64876033 0.64958678 0.65041322 0.65123967 0.65206612 0.65289256 0.65371901 0.65454545 0.6553719 0.65619835 0.65702479 0.65785124 0.65867769 0.65950413 0.66033058 0.66115702 0.66198347 0.66280992 0.66363636 0.66446281 0.66528926 0.6661157 0.66694215 0.6677686 0.66859504 0.66942149 0.67024793 0.67107438 0.67190083 0.67272727 0.67355372 0.67438017 0.67520661 0.67603306 0.6768595 0.67768595 0.6785124 0.67933884 0.68016529 0.68099174 0.68181818 0.68264463 0.68347107 0.68429752 0.68512397 0.68595041 0.68677686 0.68760331 0.68842975 0.6892562 0.69008264 0.69090909 0.69173554 0.69256198 0.69338843 0.69421488 0.69504132 0.69586777 0.69669421 0.69752066 0.69834711 0.69917355 0.7 0.70082645 0.70165289 0.70247934 0.70330579 0.70413223 0.70495868 0.70578512 0.70661157 0.70743802 0.70826446 0.70909091 0.70991736 0.7107438 0.71157025 0.71239669 0.71322314 0.71404959 0.71487603 0.71570248 0.71652893 0.71735537 0.71818182 0.71900826 0.71983471 0.72066116 0.7214876 0.72231405 0.7231405 0.72396694 0.72479339 0.72561983 0.72644628 0.72727273 0.72809917 0.72892562 0.72975207 0.73057851 0.73140496 0.7322314 0.73305785 0.7338843 0.73471074 0.73553719 0.73636364 0.73719008 0.73801653 0.73884298 0.73966942 0.74049587 0.74132231 0.74214876 0.74297521 0.74380165 0.7446281 0.74545455 0.74628099 0.74710744 0.74793388 0.74876033 0.74958678 0.75041322 0.75123967 0.75206612 0.75289256 0.75371901 0.75454545 0.7553719 0.75619835 0.75702479 0.75785124 0.75867769 0.75950413 0.76033058 0.76115702 0.76198347 0.76280992 0.76363636 0.76446281 0.76528926 0.7661157 0.76694215 0.7677686 0.76859504 0.76942149 0.77024793 0.77107438 0.77190083 0.77272727 0.77355372 0.77438017 0.77520661 0.77603306 0.7768595 0.77768595 0.7785124 0.77933884 0.78016529 0.78099174 0.78181818 0.78264463 0.78347107 0.78429752 0.78512397 0.78595041 0.78677686 0.78760331 0.78842975 0.7892562 0.79008264 0.79090909 0.79173554 0.79256198 0.79338843 0.79421488 0.79504132 0.79586777 0.79669421 0.79752066 0.79834711 0.79917355 0.8 0.80082645 0.80165289 0.80247934 0.80330579 0.80413223 0.80495868 0.80578512 0.80661157 0.80743802 0.80826446 0.80909091 0.80991736 0.8107438 0.81157025 0.81239669 0.81322314 0.81404959 0.81487603 0.81570248 0.81652893 0.81735537 0.81818182 0.81900826 0.81983471 0.82066116 0.8214876 0.82231405 0.8231405 0.82396694 0.82479339 0.82561983 0.82644628 0.82727273 0.82809917 0.82892562 0.82975207 0.83057851 0.83140496 0.8322314 0.83305785 0.8338843 0.83471074 0.83553719 0.83636364 0.83719008 0.83801653 0.83884298 0.83966942 0.84049587 0.84132231 0.84214876 0.84297521 0.84380165 0.8446281 0.84545455 0.84628099 0.84710744 0.84793388 0.84876033 0.84958678 0.85041322 0.85123967 0.85206612 0.85289256 0.85371901 0.85454545 0.8553719 0.85619835 0.85702479 0.85785124 0.85867769 0.85950413 0.86033058 0.86115702 0.86198347 0.86280992 0.86363636 0.86446281 0.86528926 0.8661157 0.86694215 0.8677686 0.86859504 0.86942149 0.87024793 0.87107438 0.87190083 0.87272727 0.87355372 0.87438017 0.87520661 0.87603306 0.8768595 0.87768595 0.8785124 0.87933884 0.88016529 0.88099174 0.88181818 0.88264463 0.88347107 0.88429752 0.88512397 0.88595041 0.88677686 0.88760331 0.88842975 0.8892562 0.89008264 0.89090909 0.89173554 0.89256198 0.89338843 0.89421488 0.89504132 0.89586777 0.89669421 0.89752066 0.89834711 0.89917355 0.9 0.90082645 0.90165289 0.90247934 0.90330579 0.90413223 0.90495868 0.90578512 0.90661157 0.90743802 0.90826446 0.90909091 0.90991736 0.9107438 0.91157025 0.91239669 0.91322314 0.91404959 0.91487603 0.91570248 0.91652893 0.91735537 0.91818182 0.91900826 0.91983471 0.92066116 0.9214876 0.92231405 0.9231405 0.92396694 0.92479339 0.92561983 0.92644628 0.92727273 0.92809917 0.92892562 0.92975207 0.93057851 0.93140496 0.9322314 0.93305785 0.9338843 0.93471074 0.93553719 0.93636364 0.93719008 0.93801653 0.93884298 0.93966942 0.94049587 0.94132231 0.94214876 0.94297521 0.94380165 0.9446281 0.94545455 0.94628099 0.94710744 0.94793388 0.94876033 0.94958678 0.95041322 0.95123967 0.95206612 0.95289256 0.95371901 0.95454545 0.9553719 0.95619835 0.95702479 0.95785124 0.95867769 0.95950413 0.96033058 0.96115702 0.96198347 0.96280992 0.96363636 0.96446281 0.96528926 0.9661157 0.96694215 0.9677686 0.96859504 0.96942149 0.97024793 0.97107438 0.97190083 0.97272727 0.97355372 0.97438017 0.97520661 0.97603306 0.9768595 0.97768595 0.9785124 0.97933884 0.98016529 0.98099174 0.98181818 0.98264463 0.98347107 0.98429752 0.98512397 0.98595041 0.98677686 0.98760331 0.98842975 0.9892562 0.99008264 0.99090909 0.99173554 0.99256198 0.99338843 0.99421488 0.99504132 0.99586777 0.99669421 0.99752066 0.99834711 0.99917355 1 1 1 1 1 1
  spline S2 degree 5 poles (52.4636, 56.3547) (52.4851, 56.3505) (52.5279, 56.3414) (52.5917, 56.3258) (52.6758, 56.3012) (52.7792, 56.2647) (52.8808, 56.2229) (52.9805, 56.1765) (53.0781, 56.1258) (53.1733, 56.071) (53.2656, 56.0118) (53.3547, 55.9481) (53.44, 55.8796) (53.5213, 55.8063) (53.5981, 55.7283) (53.6705, 55.6458) (53.7382, 55.5591) (53.8011, 55.4688) (53.859, 55.3752) (53.9116, 55.2786) (53.9586, 55.1794) (53.9996, 55.0779) (54.0345, 54.9743) (54.0631, 54.8688) (54.0858, 54.7619) (54.103, 54.6536) (54.1149, 54.5443) (54.1219, 54.4344) (54.1239, 54.3241) (54.1206, 54.214) (54.1113, 54.1044) (54.0953, 53.996) (54.0723, 53.889) (54.0422, 53.7839) (54.0052, 53.6808) (53.9622, 53.5798) (53.9142, 53.4809) (53.8624, 53.3839) (53.8079, 53.2886) (53.7516, 53.1946) (53.6943, 53.1013) (53.6367, 53.0085) (53.5791, 52.9156) (53.5219, 52.8225) (53.4651, 52.729) (53.4087, 52.6351) (53.3524, 52.5411) (53.2962, 52.4471) (53.2399, 52.3531) (53.1835, 52.2592) (53.127, 52.1655) (53.0704, 52.0718) (53.0138, 51.9782) (52.9573, 51.8845) (52.9008, 51.7907) (52.8444, 51.6969) (52.7879, 51.6031) (52.7315, 51.5092) (52.675, 51.4154) (52.6184, 51.3216) (52.5619, 51.2279) (52.5055, 51.1341) (52.4491, 51.0403) (52.3928, 50.9465) (52.3364, 50.8527) (52.28, 50.759) (52.2234, 50.6652) (52.1666, 50.5715) (52.1097, 50.4778) (52.0528, 50.3841) (51.9962, 50.2903) (51.9399, 50.1965) (51.8841, 50.1026) (51.8286, 50.0087) (51.7731, 49.9147) (51.7171, 49.8209) (51.6602, 49.7272) (51.6022, 49.6336) (51.5434, 49.5402) (51.4847, 49.4468) (51.4272, 49.3531) (51.3719, 49.2592) (51.319, 49.1647) (51.2681, 49.07) (51.2169, 48.9753) (51.1631, 48.8811) (51.1042, 48.7877) (51.0395, 48.6953) (50.9699, 48.6037) (50.8997, 48.5121) (50.8351, 48.4195) (50.7826, 48.3249) (50.7479, 48.2276) (50.7346, 48.1275) (50.7426, 48.0254) (50.769, 47.9227) (50.8096, 47.8207) (50.8593, 47.7209) (50.9141, 47.6239) (50.9712, 47.5296) (51.0289, 47.4371) (51.0864, 47.3455) (51.1436, 47.2539) (51.2004, 47.1614) (51.2569, 47.0679) (51.3133, 46.9737) (51.3696, 46.8791) (51.4259, 46.7844) (51.4823, 46.6901) (51.5388, 46.5963) (51.5954, 46.5027) (51.652, 46.4094) (51.7087, 46.3161) (51.7653, 46.2226) (51.8219, 46.1289) (51.8784, 46.0351) (51.9349, 45.9412) (51.9914, 45.8473) (52.0479, 45.7535) (52.1044, 45.6597) (52.1609, 45.566) (52.2174, 45.4723) (52.274, 45.3787) (52.3306, 45.285) (52.3872, 45.1913) (52.4438, 45.0976) (52.5004, 45.0039) (52.557, 44.9102) (52.6135, 44.8164) (52.6701, 44.7227) (52.7266, 44.629) (52.7832, 44.5353) (52.8398, 44.4416) (52.8964, 44.3479) (52.953, 44.2542) (53.0096, 44.1605) (53.0662, 44.0667) (53.1226, 43.973) (53.179, 43.8792) (53.2354, 43.7854) (53.2919, 43.6916) (53.3484, 43.5979) (53.4051, 43.5041) (53.4619, 43.4105) (53.5187, 43.3169) (53.5755, 43.2232) (53.632, 43.1295) (53.6878, 43.0354) (53.7425, 42.9408) (53.7955, 42.8452) (53.8459, 42.7481) (53.893, 42.6492) (53.9359, 42.5481) (53.9737, 42.4448) (54.0056, 42.3394) (54.0309, 42.2324) (54.0489, 42.1241) (54.0595, 42.0151) (54.0628, 41.9057) (54.0593, 41.7963) (54.0498, 41.6872) (54.035, 41.5784) (54.0157, 41.4702) (53.9921, 41.3629) (53.9643, 41.2567) (53.9318, 41.152) (53.8941, 41.0493) (53.8508, 40.9489) (53.8015, 40.8512) (53.7464, 40.7564) (53.6855, 40.665) (53.6193, 40.5771) (53.5483, 40.4929) (53.4728, 40.4128) (53.3932, 40.337) (53.3099, 40.2656) (53.2229, 40.199) (53.1325, 40.1373) (53.0389, 40.0805) (52.9423, 40.0289) (52.8431, 39.9824) (52.7414, 39.9411) (52.6375, 39.9051) (52.5319, 39.8747) (52.4247, 39.8502) (52.3164, 39.8321) (52.2074, 39.8206) (52.0979, 39.816) (51.9884, 39.8182) (51.8791, 39.827) (51.7705, 39.8419) (51.6627, 39.8624) (51.5561, 39.8881) (51.4509, 39.9186) (51.3473, 39.954) (51.2456, 39.9942) (51.1459, 40.0395) (51.0487, 40.0902) (50.9544, 40.1464) (50.8635, 40.2082) (50.7767, 40.2756) (50.6945, 40.3483) (50.6172, 40.426) (50.5449, 40.5082) (50.4771, 40.5942) (50.4132, 40.6832) (50.3524, 40.7744) (50.2938, 40.8671) (50.2366, 40.9605) (50.1802, 41.0544) (50.1243, 41.1485) (50.0684, 41.2425) (50.0125, 41.3365) (49.9563, 41.4304) (49.8999, 41.5242) (49.8434, 41.618) (49.7868, 41.7117) (49.7302, 41.8055) (49.6737, 41.8993) (49.6173, 41.9931) (49.5609, 42.0869) (49.5046, 42.1807) (49.4483, 42.2746) (49.392, 42.3684) (49.3356, 42.4622) (49.2792, 42.556) (49.2227, 42.6498) (49.1662, 42.7436) (49.1098, 42.8374) (49.0533, 42.9311) (48.9968, 43.0249) (48.9403, 43.1187) (48.8838, 43.2125) (48.8273, 43.3062) (48.7709, 43.4) (48.7144, 43.4938) (48.658, 43.5876) (48.6015, 43.6814) (48.5451, 43.7752) (48.4886, 43.869) (48.4322, 43.9628) (48.3757, 44.0566) (48.3193, 44.1503) (48.2628, 44.2441) (48.2064, 44.3379) (48.1499, 44.4317) (48.0935, 44.5255) (48.037, 44.6193) (47.9805, 44.7131) (47.924, 44.8068) (47.8675, 44.9006) (47.811, 44.9943) (47.7545, 45.0881) (47.698, 45.1819) (47.6415, 45.2757) (47.5851, 45.3695) (47.5286, 45.4633) (47.472, 45.557) (47.4155, 45.6507) (47.359, 45.7445) (47.3025, 45.8382) (47.246, 45.932) (47.1895, 46.0259) (47.1331, 46.1197) (47.0766, 46.2136) (47.0201, 46.3074) (46.9636, 46.4011) (46.9069, 46.4947) (46.8502, 46.5881) (46.7934, 46.6816) (46.7366, 46.7751) (46.6801, 46.869) (46.6243, 46.9634) (46.5698, 47.0587) (46.5176, 47.1551) (46.4688, 47.2532) (46.4245, 47.353) (46.3855, 47.4549) (46.3527, 47.5589) (46.3263, 47.6649) (46.3061, 47.7727) (46.2922, 47.8818) (46.2843, 47.9918) (46.2826, 48.1022) (46.2873, 48.2123) (46.2989, 48.3216) (46.3178, 48.4294) (46.3441, 48.5355) (46.3777, 48.6394) (46.4178, 48.7412) (46.4635, 48.8408) (46.5136, 48.9386) (46.5667, 49.0347) (46.6218, 49.1297) (46.6781, 49.2237) (46.7349, 49.3172) (46.7918, 49.4105) (46.8486, 49.5038) (46.9052, 49.5973) (46.9616, 49.6911) (47.0178, 49.7851) (47.074, 49.8792) (47.1301, 49.9732) (47.1863, 50.0672) (47.2427, 50.1611) (47.2991, 50.2549) (47.3555, 50.3487) (47.412, 50.4424) (47.4684, 50.5362) (47.5248, 50.63) (47.5812, 50.7238) (47.6375, 50.8177) (47.6939, 50.9116) (47.7502, 51.0054) (47.8065, 51.0993) (47.8628, 51.1932) (47.9191, 51.287) (47.9755, 51.3809) (48.0318, 51.4747) (48.0881, 51.5686) (48.1444, 51.6625) (48.2007, 51.7563) (48.257, 51.8502) (48.3133, 51.9441) (48.3697, 52.0379) (48.426, 52.1318) (48.4823, 52.2256) (48.5387, 52.3195) (48.5951, 52.4133) (48.6515, 52.5071) (48.7078, 52.6009) (48.7642, 52.6947) (48.8206, 52.7885) (48.877, 52.8824) (48.9334, 52.9762) (48.9897, 53.07) (49.0461, 53.1638) (49.1024, 53.2577) (49.1588, 53.3515) (49.2151, 53.4454) (49.2715, 53.5392) (49.3279, 53.633) (49.3844, 53.7268) (49.4408, 53.8206) (49.4973, 53.9144) (49.5536, 54.0082) (49.6099, 54.1021) (49.6661, 54.1961) (49.7222, 54.29) (49.7784, 54.384) (49.8348, 54.4778) (49.8914, 54.5715) (49.9482, 54.6651) (50.0052, 54.7585) (50.0621, 54.852) (50.1186, 54.9457) (50.1746, 55.0398) (50.2299, 55.1343) (50.285, 55.2289) (50.3406, 55.3233) (50.3976, 55.4169) (50.4571, 55.5088) (50.5202, 55.5984) (50.5877, 55.6847) (50.6599, 55.7673) (50.737, 55.8454) (50.8188, 55.9187) (50.9049, 55.9869) (50.995, 56.0496) (51.0885, 56.107) (51.1851, 56.1591) (51.2843, 56.2058) (51.3856, 56.2474) (51.4889, 56.2839) (51.5938, 56.3152) (51.7002, 56.3413) (51.808, 56.3619) (51.9168, 56.3769) (52.0265, 56.3859) (52.1365, 56.3886) (52.2464, 56.3847) (52.3339, 56.3761) (52.3989, 56.3666) (52.4421, 56.3589) (52.4636, 56.3547) knots 0 0 0 0 0 0 0.00263158 0.00526316 0.00789474 0.01052632 0.01315789 0.01578947 0.01842105 0.02105263 0.02368421 0.02631579 0.02894737 0.03157895 0.03421053 0.03684211 0.03947368 0.04210526 0.04473684 0.04736842 0.05 0.05263158 0.05526316 0.05789474 0.06052632 0.06315789 0.06578947 0.06842105 0.07105263 0.07368421 0.07631579 0.07894737 0.08157895 0.08421053 0.08684211 0.08947368 0.09210526 0.09473684 0.09736842 0.1 0.10263158 0.10526316 0.10789474 0.11052632 0.11315789 0.11578947 0.11842105 0.12105263 0.12368421 0.12631579 0.12894737 0.13157895 0.13421053 0.13684211 0.13947368 0.14210526 0.14473684 0.14736842 0.15 0.15263158 0.15526316 0.15789474 0.16052632 0.16315789 0.16578947 0.16842105 0.17105263 0.17368421 0.17631579 0.17894737 0.18157895 0.18421053 0.18684211 0.18947368 0.19210526 0.19473684 0.19736842 0.2 0.20263158 0.20526316 0.20789474 0.21052632 0.21315789 0.21578947 0.21842105 0.22105263 0.22368421 0.22631579 0.22894737 0.23157895 0.23421053 0.23684211 0.23947368 0.24210526 0.24473684 0.24736842 0.25 0.25263158 0.25526316 0.25789474 0.26052632 0.26315789 0.26578947 0.26842105 0.27105263 0.27368421 0.27631579 0.27894737 0.28157895 0.28421053 0.28684211 0.28947368 0.29210526 0.29473684 0.29736842 0.3 0.30263158 0.30526316 0.30789474 0.31052632 0.31315789 0.31578947 0.31842105 0.32105263 0.32368421 0.32631579 0.32894737 0.33157895 0.33421053 0.33684211 0.33947368 0.34210526 0.34473684 0.34736842 0.35 0.35263158 0.35526316 0.35789474 0.36052632 0.36315789 0.36578947 0.36842105 0.37105263 0.37368421 0.37631579 0.37894737 0.38157895 0.38421053 0.38684211 0.38947368 0.39210526 0.39473684 0.39736842 0.4 0.40263158 0.40526316 0.40789474 0.41052632 0.41315789 0.41578947 0.41842105 0.42105263 0.42368421 0.42631579 0.42894737 0.43157895 0.43421053 0.43684211 0.43947368 0.44210526 0.44473684 0.44736842 0.45 0.45263158 0.45526316 0.45789474 0.46052632 0.46315789 0.46578947 0.46842105 0.47105263 0.47368421 0.47631579 0.47894737 0.48157895 0.48421053 0.48684211 0.48947368 0.49210526 0.49473684 0.49736842 0.5 0.50263158 0.50526316 0.50789474 0.51052632 0.51315789 0.51578947 0.51842105 0.52105263 0.52368421 0.52631579 0.52894737 0.53157895 0.53421053 0.53684211 0.53947368 0.54210526 0.54473684 0.54736842 0.55 0.55263158 0.55526316 0.55789474 0.56052632 0.56315789 0.56578947 0.56842105 0.57105263 0.57368421 0.57631579 0.57894737 0.58157895 0.58421053 0.58684211 0.58947368 0.59210526 0.59473684 0.59736842 0.6 0.60263158 0.60526316 0.60789474 0.61052632 0.61315789 0.61578947 0.61842105 0.62105263 0.62368421 0.62631579 0.62894737 0.63157895 0.63421053 0.63684211 0.63947368 0.64210526 0.64473684 0.64736842 0.65 0.65263158 0.65526316 0.65789474 0.66052632 0.66315789 0.66578947 0.66842105 0.67105263 0.67368421 0.67631579 0.67894737 0.68157895 0.68421053 0.68684211 0.68947368 0.69210526 0.69473684 0.69736842 0.7 0.70263158 0.70526316 0.70789474 0.71052632 0.71315789 0.71578947 0.71842105 0.72105263 0.72368421 0.72631579 0.72894737 0.73157895 0.73421053 0.73684211 0.73947368 0.74210526 0.74473684 0.74736842 0.75 0.75263158 0.75526316 0.75789474 0.76052632 0.76315789 0.76578947 0.76842105 0.77105263 0.77368421 0.77631579 0.77894737 0.78157895 0.78421053 0.78684211 0.78947368 0.79210526 0.79473684 0.79736842 0.8 0.80263158 0.80526316 0.80789474 0.81052632 0.81315789 0.81578947 0.81842105 0.82105263 0.82368421 0.82631579 0.82894737 0.83157895 0.83421053 0.83684211 0.83947368 0.84210526 0.84473684 0.84736842 0.85 0.85263158 0.85526316 0.85789474 0.86052632 0.86315789 0.86578947 0.86842105 0.87105263 0.87368421 0.87631579 0.87894737 0.88157895 0.88421053 0.88684211 0.88947368 0.89210526 0.89473684 0.89736842 0.9 0.90263158 0.90526316 0.90789474 0.91052632 0.91315789 0.91578947 0.91842105 0.92105263 0.92368421 0.92631579 0.92894737 0.93157895 0.93421053 0.93684211 0.93947368 0.94210526 0.94473684 0.94736842 0.95 0.95263158 0.95526316 0.95789474 0.96052632 0.96315789 0.96578947 0.96842105 0.97105263 0.97368421 0.97631579 0.97894737 0.98157895 0.98421053 0.98684211 0.98947368 0.99210526 0.99473684 0.99736842 1 1 1 1 1 1